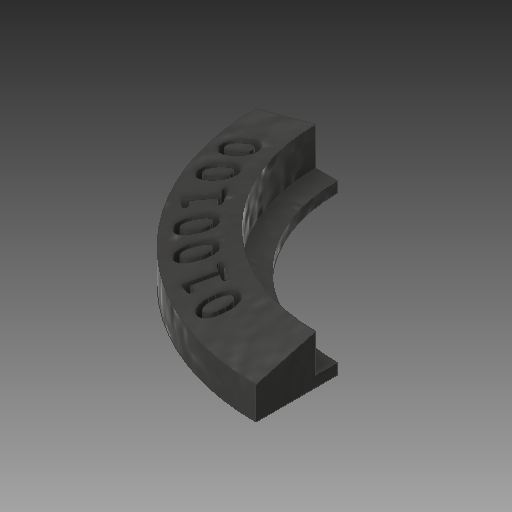
# Autodesk Inventor part: Mentor-Code ring
Saved by Autodesk Inventor 2017 (Build 210142000, 142)
## iProperties
Created: 2016-02-20
Part Number: Mentor-Code ring
Material: Generic
Document SubType Name: Modeling
Designer: RoksBot
Density: 1 g/cm^3
Appearance: Fine Textured - Black
Author: RoksBot
Autodesk Inventor part; units mm, degrees
ref_plane "YZ Plane" through (0, 0, 0) normal (1, 0, 0) x (0, 1, 0)
ref_plane "XZ Plane" through (0, 0, 0) normal (0, 1, 0) x (-1, 0, 0)
ref_plane "XY Plane" through (0, 0, 0) normal (0, 0, 1) x (1, 0, 0)
sketch "Sketch1" plane through (0, 0, 0) normal (0, 0, 1) x (1, 0, 0)
  line L0 (0, 0) -> (0, 8.6646) construction
  line L1 (20.9931, 1.27) -> (20.9931, 5.715)
  line L2 (20.9931, 5.715) -> (27.9781, 3.81)
  line L3 (27.9781, 3.81) -> (27.9781, 0)
  line L4 (27.9781, 0) -> (20.9931, 0)
  line L5 (20.9931, 1.27) -> (18.4531, 1.27)
  line L6 (18.4531, 1.27) -> (18.4531, 0)
  line L7 (18.4531, 0) -> (20.9931, 0)
  dimension "d0" = 20.9931
  dimension "d1" = 4.445
  dimension "d2" = 1.27
  dimension "d3" = 2.54
  dimension "d4" = 3.81
  dimension "d5" = 6.985
  constraints: 16 end point, 2 parallel, 2 perpendicular, 2 vertical, 1 horizontal, 1 horizontal alignment
  measures "d0" distance between parallel lines of L0 L1
  measures "d1" distance from line of L5 L1.end
  measures "d2" distance of L5.end L6.end
  measures "d3" distance between parallel lines of L1 L6
  measures "d4" distance of L2.end L3.end
  measures "d5" distance between parallel lines of L1 L3
revolve "Revolution1" add sketch "Sketch1" angle 360 about axis through (0, 0, 0) along (0, 1, 0)
sketch "Sketch2" plane through (0, 1.27, 0) normal (0, 1, 0) x (1, 0, 0)
  circle A0 centre (0, 0) radius 18.4531 projected
  circle A1 centre (0, 0) radius 27.9781 projected
  circle A2 centre (0, 0) radius 20.9931 projected
  circle A3 centre (0, 0) radius 22.8981
  line L0 (-10.8255, -22.716) -> (-10.574, -22.1086)
  spline S0 degree 2 poles (-10.574, -22.1086) (-10.3492, -21.5656) (-9.3131, -20.8338) (-8.7303, -21.0751) knots 0 0 0 1 2 2 2
  spline S1 degree 2 poles (-8.7303, -21.0751) (-8.3928, -21.2148) (-8.0515, -21.7011) (-7.9663, -22.6671) (-8.1505, -23.1119) knots 0 0 0 1 2 3 3 3
  line L1 (-8.1505, -23.1119) -> (-8.4019, -23.7193)
  spline S2 degree 2 poles (-8.4019, -23.7193) (-8.6254, -24.2592) (-9.6597, -24.9954) (-10.2426, -24.7541) knots 0 0 0 1 2 2 2
  spline S3 degree 2 poles (-10.2426, -24.7541) (-10.5769, -24.6156) (-10.9195, -24.1324) (-11.0109, -23.1639) (-10.8255, -22.716) knots 0 0 0 1 2 3 3 3
  spline S4 degree 2 poles (-10.2702, -22.9459) (-10.4581, -23.3999) (-10.3463, -23.8415) knots 0 0 0 1 1 1
  spline S5 degree 2 poles (-10.3463, -23.8415) (-10.2796, -24.0883) (-10.0188, -24.1963) knots 0 0 0 1 1 1
  spline S6 degree 2 poles (-10.0188, -24.1963) (-9.7642, -24.3017) (-9.5196, -24.1622) knots 0 0 0 1 1 1
  spline S7 degree 2 poles (-9.5196, -24.1622) (-9.1477, -23.9496) (-8.9572, -23.4894) knots 0 0 0 1 1 1
  line L2 (-8.9572, -23.4894) -> (-8.7057, -22.882)
  spline S8 degree 2 poles (-8.7057, -22.882) (-8.5165, -22.4249) (-8.6327, -21.9851) knots 0 0 0 1 1 1
  spline S9 degree 2 poles (-8.6327, -21.9851) (-8.6963, -21.7396) (-8.9601, -21.6304) knots 0 0 0 1 1 1
  spline S10 degree 2 poles (-8.9601, -21.6304) (-9.2117, -21.5262) (-9.4563, -21.6657) knots 0 0 0 1 1 1
  spline S11 degree 2 poles (-9.4563, -21.6657) (-9.8282, -21.8783) (-10.0187, -22.3385) knots 0 0 0 1 1 1
  line L3 (-10.0187, -22.3385) -> (-10.2702, -22.9459)
  line L4 (-14.2533, -22.6851) -> (-12.5348, -19.8791)
  line L5 (-12.5348, -19.8791) -> (-13.0529, -19.5618)
  spline S12 degree 2 poles (-13.0529, -19.5618) (-13.2455, -19.4439) (-13.3173, -19.2052) (-13.2462, -19.0891) knots 0 0 0 1 2 2 2
  spline S13 degree 2 poles (-13.2462, -19.0891) (-13.1752, -18.973) (-12.9316, -18.9314) (-12.7391, -19.0493) knots 0 0 0 1 2 2 2
  line L6 (-12.7391, -19.0493) -> (-11.1903, -19.9978)
  spline S14 degree 2 poles (-11.1903, -19.9978) (-10.9977, -20.1157) (-10.9259, -20.3544) (-10.997, -20.4705) knots 0 0 0 1 2 2 2
  spline S15 degree 2 poles (-10.997, -20.4705) (-11.0681, -20.5866) (-11.3116, -20.6282) (-11.5041, -20.5103) knots 0 0 0 1 2 2 2
  line L7 (-11.5041, -20.5103) -> (-12.0223, -20.193)
  line L8 (-12.0223, -20.193) -> (-13.3315, -22.3307)
  line L9 (-13.3315, -22.3307) -> (-12.8, -22.4927)
  spline S16 degree 2 poles (-12.8, -22.4927) (-12.6705, -22.5292) (-12.6167, -22.5622) knots 0 0 0 1 1 1
  spline S17 degree 2 poles (-12.6167, -22.5622) (-12.5176, -22.6229) (-12.4714, -22.8653) (-12.5408, -22.9785) knots 0 0 0 1 2 2 2
  spline S18 degree 2 poles (-12.5408, -22.9785) (-12.6032, -23.0805) (-12.7791, -23.1324) (-12.9739, -23.0754) knots 0 0 0 1 2 2 2
  line L10 (-12.9739, -23.0754) -> (-14.2533, -22.6851)
  line L11 (-17.3125, -18.2616) -> (-16.8857, -17.7615)
  spline S19 degree 2 poles (-16.8857, -17.7615) (-16.5042, -17.3145) (-15.2927, -16.9385) (-14.8129, -17.3481) knots 0 0 0 1 2 2 2
  spline S20 degree 2 poles (-14.8129, -17.3481) (-14.5351, -17.5852) (-14.3607, -18.1531) (-14.578, -19.0982) (-14.8905, -19.4644) knots 0 0 0 1 2 3 3 3
  line L12 (-14.8905, -19.4644) -> (-15.3173, -19.9644)
  spline S21 degree 2 poles (-15.3173, -19.9644) (-15.6967, -20.4089) (-16.9077, -20.7896) (-17.3876, -20.3801) knots 0 0 0 1 2 2 2
  spline S22 degree 2 poles (-17.3876, -20.3801) (-17.6629, -20.1451) (-17.8394, -19.5797) (-17.6272, -18.6303) (-17.3125, -18.2616) knots 0 0 0 1 2 3 3 3
  spline S23 degree 2 poles (-16.8553, -18.6517) (-17.1744, -19.0255) (-17.2044, -19.4801) knots 0 0 0 1 1 1
  spline S24 degree 2 poles (-17.2044, -19.4801) (-17.2172, -19.7354) (-17.0025, -19.9186) knots 0 0 0 1 1 1
  spline S25 degree 2 poles (-17.0025, -19.9186) (-16.7929, -20.0975) (-16.5171, -20.0404) knots 0 0 0 1 1 1
  spline S26 degree 2 poles (-16.5171, -20.0404) (-16.0978, -19.9531) (-15.7744, -19.5743) knots 0 0 0 1 1 1
  line L13 (-15.7744, -19.5743) -> (-15.3477, -19.0742)
  spline S27 degree 2 poles (-15.3477, -19.0742) (-15.0265, -18.6979) (-15.0012, -18.2437) knots 0 0 0 1 1 1
  spline S28 degree 2 poles (-15.0012, -18.2437) (-14.9858, -17.9905) (-15.203, -17.8052) knots 0 0 0 1 1 1
  spline S29 degree 2 poles (-15.203, -17.8052) (-15.4101, -17.6284) (-15.6859, -17.6855) knots 0 0 0 1 1 1
  spline S30 degree 2 poles (-15.6859, -17.6855) (-16.1052, -17.7729) (-16.4286, -18.1517) knots 0 0 0 1 1 1
  line L14 (-16.4286, -18.1517) -> (-16.8553, -18.6517)
  line L15 (-19.9549, -15.33) -> (-19.4552, -14.9028)
  spline S31 degree 2 poles (-19.4552, -14.9028) (-19.0084, -14.521) (-17.7531, -14.339) (-17.3432, -14.8185) knots 0 0 0 1 2 2 2
  spline S32 degree 2 poles (-17.3432, -14.8185) (-17.1059, -15.0962) (-17.0224, -15.6844) (-17.3849, -16.5839) (-17.7508, -16.8967) knots 0 0 0 1 2 3 3 3
  line L16 (-17.7508, -16.8967) -> (-18.2505, -17.3238)
  spline S33 degree 2 poles (-18.2505, -17.3238) (-18.6947, -17.7035) (-19.9504, -17.8902) (-20.3603, -17.4107) knots 0 0 0 1 2 2 2
  spline S34 degree 2 poles (-20.3603, -17.4107) (-20.5955, -17.1356) (-20.6815, -16.5495) (-20.3234, -15.645) (-19.9549, -15.33) knots 0 0 0 1 2 3 3 3
  spline S35 degree 2 poles (-19.5644, -15.7868) (-19.9379, -16.1061) (-20.0386, -16.5504) knots 0 0 0 1 1 1
  spline S36 degree 2 poles (-20.0386, -16.5504) (-20.0912, -16.8006) (-19.9078, -17.0151) knots 0 0 0 1 1 1
  spline S37 degree 2 poles (-19.9078, -17.0151) (-19.7288, -17.2246) (-19.4475, -17.2113) knots 0 0 0 1 1 1
  spline S38 degree 2 poles (-19.4475, -17.2113) (-19.0196, -17.1906) (-18.641, -16.867) knots 0 0 0 1 1 1
  line L17 (-18.641, -16.867) -> (-18.1413, -16.4399)
  spline S39 degree 2 poles (-18.1413, -16.4399) (-17.7653, -16.1184) (-17.6692, -15.6738) knots 0 0 0 1 1 1
  spline S40 degree 2 poles (-17.6692, -15.6738) (-17.6145, -15.4261) (-17.8, -15.209) knots 0 0 0 1 1 1
  spline S41 degree 2 poles (-17.8, -15.209) (-17.977, -15.0021) (-18.2582, -15.0154) knots 0 0 0 1 1 1
  spline S42 degree 2 poles (-18.2582, -15.0154) (-18.6861, -15.0361) (-19.0647, -15.3597) knots 0 0 0 1 1 1
  line L18 (-19.0647, -15.3597) -> (-19.5644, -15.7868)
  line L19 (-22.9954, -13.747) -> (-20.1908, -12.0264)
  line L20 (-20.1908, -12.0264) -> (-20.5085, -11.5085)
  spline S43 degree 2 poles (-20.5085, -11.5085) (-20.6266, -11.316) (-20.5823, -11.0707) (-20.4662, -10.9995) knots 0 0 0 1 2 2 2
  spline S44 degree 2 poles (-20.4662, -10.9995) (-20.3502, -10.9283) (-20.1143, -11.0017) (-19.9962, -11.1942) knots 0 0 0 1 2 2 2
  line L21 (-19.9962, -11.1942) -> (-19.0465, -12.7423)
  spline S45 degree 2 poles (-19.0465, -12.7423) (-18.9285, -12.9347) (-18.9727, -13.18) (-19.0888, -13.2512) knots 0 0 0 1 2 2 2
  spline S46 degree 2 poles (-19.0888, -13.2512) (-19.2048, -13.3224) (-19.4407, -13.249) (-19.5588, -13.0565) knots 0 0 0 1 2 2 2
  line L22 (-19.5588, -13.0565) -> (-19.8765, -12.5386)
  line L23 (-19.8765, -12.5386) -> (-22.0133, -13.8495)
  line L24 (-22.0133, -13.8495) -> (-21.6131, -14.235)
  spline S47 degree 2 poles (-21.6131, -14.235) (-21.5143, -14.3263) (-21.4813, -14.3801) knots 0 0 0 1 1 1
  spline S48 degree 2 poles (-21.4813, -14.3801) (-21.4205, -14.4791) (-21.4894, -14.7161) (-21.6026, -14.7856) knots 0 0 0 1 2 2 2
  spline S49 degree 2 poles (-21.6026, -14.7856) (-21.7045, -14.8481) (-21.8847, -14.8146) (-22.0325, -14.6754) knots 0 0 0 1 2 2 2
  line L25 (-22.0325, -14.6754) -> (-22.9954, -13.747)
  line L26 (-23.7142, -8.4169) -> (-23.107, -8.165)
  spline S50 degree 2 poles (-23.107, -8.165) (-22.5641, -7.9398) (-21.314, -8.1544) (-21.0722, -8.7371) knots 0 0 0 1 2 2 2
  spline S51 degree 2 poles (-21.0722, -8.7371) (-20.9323, -9.0745) (-21.0346, -9.6597) (-21.6571, -10.4033) (-22.1018, -10.5878) knots 0 0 0 1 2 3 3 3
  line L27 (-22.1018, -10.5878) -> (-22.709, -10.8397)
  spline S52 degree 2 poles (-22.709, -10.8397) (-23.2488, -11.0636) (-24.5007, -10.8533) (-24.7425, -10.2706) knots 0 0 0 1 2 2 2
  spline S53 degree 2 poles (-24.7425, -10.2706) (-24.8811, -9.9363) (-24.7819, -9.3524) (-24.1619, -8.6027) (-23.7142, -8.4169) knots 0 0 0 1 2 3 3 3
  spline S54 degree 2 poles (-23.4839, -8.972) (-23.9378, -9.1603) (-24.1708, -9.5518) knots 0 0 0 1 1 1
  spline S55 degree 2 poles (-24.1708, -9.5518) (-24.2981, -9.7735) (-24.1899, -10.0342) knots 0 0 0 1 1 1
  spline S56 degree 2 poles (-24.1899, -10.0342) (-24.0843, -10.2887) (-23.8127, -10.363) knots 0 0 0 1 1 1
  spline S57 degree 2 poles (-23.8127, -10.363) (-23.3993, -10.4755) (-22.9393, -10.2846) knots 0 0 0 1 1 1
  line L28 (-22.9393, -10.2846) -> (-22.3321, -10.0327)
  spline S58 degree 2 poles (-22.3321, -10.0327) (-21.8751, -9.8431) (-21.6465, -9.4499) knots 0 0 0 1 1 1
  spline S59 degree 2 poles (-21.6465, -9.4499) (-21.5179, -9.2312) (-21.6273, -8.9674) knots 0 0 0 1 1 1
  spline S60 degree 2 poles (-21.6273, -8.9674) (-21.7317, -8.716) (-22.0033, -8.6417) knots 0 0 0 1 1 1
  spline S61 degree 2 poles (-22.0033, -8.6417) (-22.4166, -8.5292) (-22.8767, -8.7201) knots 0 0 0 1 1 1
  line L29 (-22.8767, -8.7201) -> (-23.4839, -8.972)
  line L30 (-24.7386, -4.6055) -> (-24.0994, -4.4516)
  spline S62 degree 2 poles (-24.0994, -4.4516) (-23.5281, -4.314) (-22.3269, -4.7215) (-22.1792, -5.3348) knots 0 0 0 1 2 2 2
  spline S63 degree 2 poles (-22.1792, -5.3348) (-22.0937, -5.6899) (-22.2862, -6.2519) (-23.0174, -6.889) (-23.4854, -7.0017) knots 0 0 0 1 2 3 3 3
  line L31 (-23.4854, -7.0017) -> (-24.1246, -7.1556)
  spline S64 degree 2 poles (-24.1246, -7.1556) (-24.6927, -7.2924) (-25.8964, -6.8889) (-26.044, -6.2756) knots 0 0 0 1 2 2 2
  spline S65 degree 2 poles (-26.044, -6.2756) (-26.1287, -5.9237) (-25.9394, -5.3625) (-25.2099, -4.7189) (-24.7386, -4.6055) knots 0 0 0 1 2 3 3 3
  spline S66 degree 2 poles (-24.5979, -5.1897) (-25.0756, -5.3048) (-25.367, -5.6549) knots 0 0 0 1 1 1
  spline S67 degree 2 poles (-25.367, -5.6549) (-25.5274, -5.8541) (-25.4613, -6.1285) knots 0 0 0 1 1 1
  spline S68 degree 2 poles (-25.4613, -6.1285) (-25.3968, -6.3964) (-25.1401, -6.5122) knots 0 0 0 1 1 1
  spline S69 degree 2 poles (-25.1401, -6.5122) (-24.7495, -6.6879) (-24.2653, -6.5713) knots 0 0 0 1 1 1
  line L32 (-24.2653, -6.5713) -> (-23.6261, -6.4174)
  spline S70 degree 2 poles (-23.6261, -6.4174) (-23.1451, -6.3016) (-22.8578, -5.949) knots 0 0 0 1 1 1
  spline S71 degree 2 poles (-22.8578, -5.949) (-22.6966, -5.7531) (-22.7635, -5.4755) knots 0 0 0 1 1 1
  spline S72 degree 2 poles (-22.7635, -5.4755) (-22.8272, -5.2108) (-23.0839, -5.095) knots 0 0 0 1 1 1
  spline S73 degree 2 poles (-23.0839, -5.095) (-23.4745, -4.9193) (-23.9587, -5.0359) knots 0 0 0 1 1 1
  line L33 (-23.9587, -5.0359) -> (-24.5979, -5.1897)
  dimension "d7" = 1.905
  constraints: 1 centre point, 1 coincident, 1 other
  measures "d7" radial gap between concentric circles of A2 A3
extrude "Extrusion1" cut sketch "Sketch2" along normal blind 25.4 contours L6 S14 S15 L7 L8 L9 S16 S17 S18 L10 L4 L5 S12 S13 | L21 S45 S46 L22 L23 L24 S47 S48 S49 L25 L19 L20 S43 S44 | S62 S63 A3 | A3 S63 L31 S64 S65 L30 S62 | S1 L1 S2 S3 L0 S0 A3 | A3 S0 S1 | S50 S51 A3 | A3 S51 L27 S52 S53 L26 S50 | S20 L12 S21 S22 L11 S19 A3 | A3 S19 S20 | S31 S32 A3 | A3 S32 L16 S33 S34 L15 S31
sketch "Sketch3" plane through (0, 1.27, 0) normal (0, 1, 0) x (1, 0, 0)
  line L0 (0, 0) -> (-33.4384, 0)
  line L1 (-33.4384, 0) -> (-33.4384, -30.9013)
  line L2 (-33.4384, -30.9013) -> (0, -30.9013)
  line L3 (0, -30.9013) -> (0, 0)
  constraints: 8 end point, 2 parallel, 1 horizontal, 1 perpendicular
extrude "Extrusion2" cut sketch "Sketch3" along normal through all both and the other way through all keep common part
body "Solid1"
